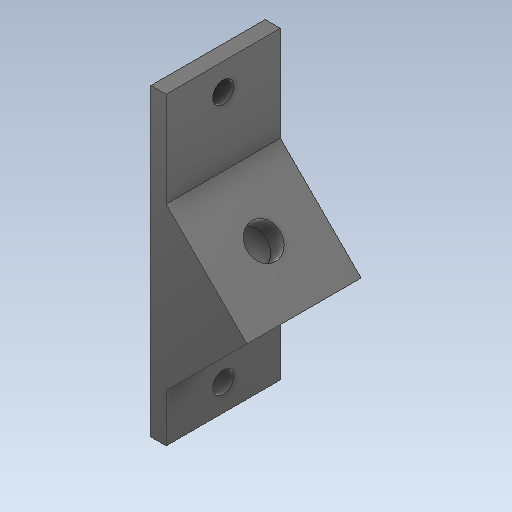
# Autodesk Inventor part: 45bracket
Saved by Autodesk Inventor 2020.2 (Build 242310000, 310)
## iProperties
Created: 2020-07-20
Part Number: 45bracket
Material: Acetal Resin, Black
Document SubType Name: Modeling
Designer: JK
Density: 1.425 g/cm^3
Appearance: Smooth - Black
Author: JK
Autodesk Inventor part; units mm, degrees
ref_plane "YZ Plane" through (0, 0, 0) normal (1, 0, 0) x (0, 1, 0)
ref_plane "XZ Plane" through (0, 0, 0) normal (0, 1, 0) x (-1, 0, 0)
sketch "Sketch6" plane through (0, 0, 0) normal (0, 0, 1) x (1, 0, 0)
  line L0 (-2, -40) -> (2, -40)
  line L1 (2, -40) -> (2, 40)
  line L2 (2, 40) -> (-2, 40)
  line L3 (-2, 40) -> (-2, -40)
  line L4 (-2, -40) -> (2, 40) construction
  line L5 (2, -40) -> (-2, 40) construction
  line L6 (2, 15) -> (23.2132, -6.2132)
  line L7 (2, 15) -> (32, 15) construction
  line L8 (23.2132, -6.2132) -> (2, -27.4264)
  line L9 (2, -27.4264) -> (2, 15)
  point P0 (0, 0)
  point P1 (2, -27.4264)
  dimension "d23" = 4
  dimension "d24" = 80
  dimension "d25" = 30
  dimension "d26" = 45
  dimension "d27" = 30
  dimension "d28" = 90
  dimension "d29" = 25
  constraints: 20 end point, 2 horizontal, 2 midpoint, 2 parallel, 2 perpendicular, 1 equal length, 1 point on line
  measures "d23" distance between parallel lines of L1 L3
  measures "d24" distance of L2.end L0.start
  measures "d25" distance of L6.start L6.end
  measures "d26" angle of L6 L7
  measures "d27" distance of L6.end L8.end
  measures "d28" angle of L6 L8
  measures "d29" distance of L1.end L6.start
extrude "Extrusion6" add sketch "Sketch6" along normal blind 30
sketch "Sketch7" plane through (2, 15, 0) normal (0.7071, 0.7071, 0) x (-0.7071, 0.7071, 0)
  circle A0 centre (-15, 15) radius 4.4
  line L0 (-30, 0) -> (-30, 30) projected
  line L1 (-30, 30) -> (0, 30) projected
  point P0 (-9.1924, 0)
  dimension "d32" = 15
  dimension "d33" = 15
  dimension "d34" = 8.8
  constraints: 1 centre point
  measures "d32" distance from line of L0 A0.centre
  measures "d33" distance from line of L1 A0.centre
  measures "d34" diameter of A0
extrude "Extrusion7" cut sketch "Sketch7" against normal blind 27.5
ref_plane "Work Plane6" through (-19.9203, -6.9203, 0) normal (0.7071, 0.7071, 0) x (-0.7071, 0.7071, 0)
sketch "Sketch8" plane through (-19.9203, -6.9203, 0) normal (0.7071, 0.7071, 0) x (-0.7071, 0.7071, 0)
  circle A0 centre (-15, 15) radius 4.4 projected
  circle A1 centre (-15, 15) radius 7
  point P0 (-9.1924, 0)
  dimension "d38" = 14
  constraints: 1 centre point, 1 coincident
  measures "d38" diameter of A1
extrude "Extrusion8" cut sketch "Sketch8" along normal blind 26 contours A0 | A1
sketch "Sketch9" plane through (2, -40, 0) normal (1, 0, 0) x (0, 0, -1)
  circle A0 centre (-15, 7) radius 2.8
  line L0 (0, 0) -> (-30, 0) projected
  line L1 (-30, 0) -> (-30, 12.5736) projected
  circle A1 centre (-15, 73) radius 2.8
  line L2 (0, 55) -> (0, 80) projected
  line L3 (0, 80) -> (-30, 80) projected
  point P0 (0, 40)
  dimension "d41" = 5.6
  dimension "d42" = 7
  dimension "d43" = 15
  dimension "d46" = 15
  dimension "d47" = 7
  constraints: 2 centre point, 1 equal radius
  measures "d41" diameter of A0
  measures "d42" distance from line of L0 A0.centre
  measures "d43" distance from line of L1 A0.centre
  measures "d46" distance from line of L2 A1.centre
  measures "d47" distance from line of L3 A1.centre
extrude "Extrusion9" cut sketch "Sketch9" against normal through all
body "Solid2"
